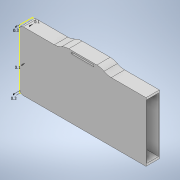
# Autodesk Inventor part: bobecase
Saved by Autodesk Inventor 2022 (Build 260153000, 153)
## iProperties
Created: 2021-10-13
Part Number: bobecase
Material: 일반
Document SubType Name: Modeling
Designer: ELEC-01
Density: 1 g/cm^3
Appearance: 기본값
Author: ELEC-01
Autodesk Inventor part; units mm, degrees
ref_plane "YZ Plane" through (0, 0, 0) normal (1, 0, 0) x (0, 1, 0)
ref_plane "XZ Plane" through (0, 0, 0) normal (0, 1, 0) x (-1, 0, 0)
sketch "스케치1" plane through (0, 0, 0) normal (0, 0, 1) x (1, 0, 0)
  line L0 (0, 0) -> (17, 0)
  line L1 (17, 0) -> (17, 8)
  line L2 (17, 8) -> (0, 8)
  line L3 (0, 8) -> (0, 0)
  line L4 (0, 4.8) -> (17, 4.8)
  line L5 (15, 8) -> (15, 0)
  dimension "d0" = 17
  dimension "d1" = 8
  dimension "d3" = 4.8
  dimension "d4" = 15
  constraints: 12 end point, 4 point on line, 3 perpendicular, 2 parallel, 1 horizontal
  measures "d0" distance of L2.end L1.end
  measures "d1" distance of L1.end L0.end
  measures "d3" distance between parallel lines of L0 L4
  measures "d4" distance between parallel lines of L3 L5
extrude "돌출1" add sketch "스케치1" along normal mid plane 1.8
sketch "스케치3" plane through (0, 0, 0.9) normal (-1, 0, 0) x (0, 0, 1)
  line L0 (-1.8, 0) -> (0, 0) projected
  line L1 (-1.8, 0) -> (-1.8, 8) projected
  line L2 (-1.7, 7.7) -> (-0.1, 7.7)
  line L3 (-0.1, 7.7) -> (-0.1, 0.3)
  line L4 (-0.1, 0.3) -> (-1.7, 0.3)
  line L5 (-1.7, 0.3) -> (-1.7, 7.7)
  line L6 (-1.8, 8) -> (0, 8) projected
  line L7 (0, 8) -> (0, 0) projected
  point P0 (-0.9, 0)
  dimension "d11" = 0.3
  dimension "d12" = 0.3
  dimension "d13" = 0.1
  dimension "d14" = 0.1
  constraints: 8 end point, 2 parallel, 1 horizontal, 1 perpendicular
  measures "d11" distance between parallel lines of L6 L2
  measures "d12" distance between parallel lines of L0 L4
  measures "d13" distance between parallel lines of L7 L3
  measures "d14" distance between parallel lines of L1 L5
sketch "스케치5" plane through (0, 0, -0.9) normal (0, 0, -1) x (-1, 0, 0)
  line L0 (0, 0) -> (0, 8) projected
  line L1 (-17, 0) -> (0, 0) projected
  line L2 (-9.9, 6.5) -> (-7.1, 6.5)
  line L3 (-7.1, 6.5) -> (-7.1, 4)
  line L4 (-7.1, 4) -> (-9.9, 4)
  line L5 (-9.9, 4) -> (-9.9, 6.5)
  line L6 (-17, 8) -> (-17, 0) projected
  line L7 (0, 8) -> (-17, 8) projected
  dimension "d21" = 2.8
  dimension "d22" = 2.5
  dimension "d24" = 1.5
  dimension "d25" = 7.1
  constraints: 8 end point, 2 parallel, 1 horizontal, 1 perpendicular
  measures "d21" distance of L3.end L4.end
  measures "d22" distance of L2.end L3.end
  measures "d24" distance between parallel lines of L7 L2
  measures "d25" distance between parallel lines of L6 L5
extrude "돌출3" add sketch "스케치5" along normal blind 1 contours L2 L3 L4 L5
sketch "스케치6" plane through (0, 0, -1.9) normal (0, 0, -1) x (-1, 0, 0)
  line L0 (-9, 5.75) -> (-8, 5.75)
  line L1 (-8, 5.75) -> (-8, 4.75)
  line L2 (-8, 4.75) -> (-9, 4.75)
  line L3 (-9, 4.75) -> (-9, 5.75)
  line L4 (-9, 5.75) -> (-8, 4.75) construction
  line L5 (-8, 5.75) -> (-9, 4.75) construction
  line L6 (0, 8) -> (-17, 8) projected
  line L7 (0, 0) -> (0, 8) projected
  point P0 (-8.5, 5.25)
  dimension "d28" = 1
  dimension "d29" = 1
  dimension "d30" = 2.75
  dimension "d31" = 8.5
  constraints: 12 end point, 2 midpoint, 2 parallel, 1 horizontal, 1 perpendicular
  measures "d28" distance of L0.end L1.end
  measures "d29" distance of L0.start L0.end
  measures "d30" distance from line of L6 point (-8.5, 5.25)
  measures "d31" distance from line of L7 point (-8.5, 5.25)
sketch "스케치7" plane through (7.1, 6.5, -0.9) normal (0, 1, 0) x (1, 0, 0)
  line L0 (0, 0) -> (0, 1) projected
  line L1 (0.1, 0.2799) -> (2.7, 0.2799)
  line L2 (2.7, 0.2799) -> (2.7, 0.7799)
  line L3 (2.7, 0.7799) -> (0.1, 0.7799)
  line L4 (0.1, 0.7799) -> (0.1, 0.2799)
  point P0 (-7.1, -0.9)
  point P1 (2.8, 0)
  dimension "d32" = 0.5
  dimension "d33" = 2.6
  dimension "d34" = 0.1
  constraints: 8 end point, 2 parallel, 1 horizontal, 1 perpendicular
  measures "d32" distance of L3.end L1.start
  measures "d33" distance of L2.end L3.end
  measures "d34" distance between parallel lines of L0 L4
extrude "돌출4" cut sketch "스케치7" against normal blind 2.49
extrude "돌출5" cut sketch "스케치6" against normal blind 0.5
sketch "스케치8" plane through (0, 8, 0.9) normal (0, 1, 0) x (1, 0, 0)
  line L0 (17, 1.8) -> (0, 1.8) projected
  line L1 (17, 0) -> (0, 0) projected
  line L2 (11, 1.8) -> (6, 1.8)
  line L3 (6, 1.8) -> (6, 0)
  line L4 (6, 0) -> (11, 0)
  line L5 (11, 0) -> (11, 1.8)
  line L6 (17, 0) -> (17, 1.8) projected
  point P0 (0, 0.9)
  point P1 (11, 0)
  dimension "d39" = 5
  dimension "d40" = 6
  constraints: 8 end point, 2 parallel, 2 point on line, 1 horizontal, 1 perpendicular
  measures "d39" distance between parallel lines of L3 L5
  measures "d40" distance between parallel lines of L6 L5
extrude "돌출6" add sketch "스케치8" along normal blind 0.5 contours L5 L1 L3 L0
sketch "스케치9" plane through (0, 0, -0.9) normal (0, 0, -1) x (-1, 0, 0)
  line L0 (-10, 8.3) -> (-7, 8.3)
  line L1 (-7, 8.3) -> (-7, 8.1)
  line L2 (-7, 8.1) -> (-10, 8.1)
  line L3 (-10, 8.1) -> (-10, 8.3)
  line L4 (-11, 8) -> (-11, 8.5) projected
  line L5 (-11, 8.5) -> (-6, 8.5) projected
  point P0 (0, 0)
  dimension "d43" = 0.2
  dimension "d44" = 3
  dimension "d45" = 1
  dimension "d46" = 0.2
  constraints: 8 end point, 2 parallel, 1 horizontal, 1 perpendicular
  measures "d43" distance of L0.end L1.end
  measures "d44" distance of L0.start L0.end
  measures "d45" distance between parallel lines of L4 L3
  measures "d46" distance between parallel lines of L5 L0
extrude "돌출7" cut sketch "스케치9" against normal blind 6
fillet "모깎기1" radius 2 4 edges at (11, 8.5, 0) (6, 8.5, 0) (11, 8, 0) (6, 8, 0)
fillet "모깎기3" radius 0.5 2 edges at (0, 0, 0) (0, 8, 0)
ref_plane "작업 평면1" through (17, 2, -0.9) normal (1, 0, 0) x (0, 0, -1)
sketch "스케치10" plane through (17, 2, -0.9) normal (1, 0, 0) x (0, 0, -1)
  line L0 (-1.7, 5.7) -> (-0.1, 5.7)
  line L1 (-0.1, 5.7) -> (-0.1, -1.7)
  line L2 (-0.1, -1.7) -> (-1.7, -1.7)
  line L3 (-1.7, -1.7) -> (-1.7, 5.7)
  line L4 (-1.8, 4) -> (-1.8, 6) projected
  line L5 (0, 4) -> (0, 0) projected
  line L6 (0, 6) -> (-1.8, 6) projected
  line L7 (-1.8, -2) -> (0, -2) projected
  point P0 (-0.9, -2)
  dimension "d52" = 0.1
  dimension "d53" = 0.1
  dimension "d54" = 0.3
  dimension "d55" = 0.3
  constraints: 8 end point, 2 parallel, 1 horizontal, 1 perpendicular
  measures "d52" distance between parallel lines of L4 L3
  measures "d53" distance between parallel lines of L5 L1
  measures "d54" distance between parallel lines of L6 L0
  measures "d55" distance between parallel lines of L7 L2
extrude "돌출8" cut sketch "스케치10" against normal blind 16.5
